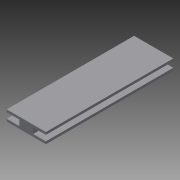
# Autodesk Inventor part: soporte fio
Saved by Autodesk Inventor 2013 (Build 170138000, 138)
## iProperties
Created: 2013-04-24
Part Number: soporte fio
Material: Generic
Document SubType Name: Modeling
Designer: otrab
Density: 1 g/cm^3
Author: otrab
Autodesk Inventor part; units mm, degrees
ref_plane "YZ Plane" through (0, 0, 0) normal (1, 0, 0) x (0, 1, 0)
ref_plane "XZ Plane" through (0, 0, 0) normal (0, 1, 0) x (-1, 0, 0)
ref_plane "XY Plane" through (0, 0, 0) normal (0, 0, 1) x (1, 0, 0)
sketch "Sketch1" plane through (0, 0, 0) normal (0, 1, 0) x (-1, 0, 0)
  line L0 (0, 0) -> (0, 1)
  line L1 (0, 1) -> (5.2, 1)
  line L2 (5.2, 1) -> (5.2, 3.3)
  line L3 (5.2, 3.3) -> (0, 3.3)
  line L4 (0, 3.3) -> (0, 4.3)
  line L5 (0, 4.3) -> (6, 4.3)
  line L6 (8, 7.1013) -> (8, -1.6755) construction
  line L7 (0, 0) -> (9, 0)
  line L8 (16, 0) -> (16, 1)
  line L9 (16, 1) -> (10.8, 1)
  line L10 (10.8, 1) -> (10.8, 3.3)
  line L11 (10.8, 3.3) -> (16, 3.3)
  line L12 (16, 3.3) -> (16, 4.3)
  line L13 (16, 4.3) -> (6, 4.3)
  line L14 (16, 0) -> (9, 0)
  dimension "d0" = 1
  dimension "d2" = 2.3
  dimension "d5" = 1
  dimension "d10" = 2.8
  dimension "d11" = 16
  dimension "d12" = 16
  constraints: 30 end point, 6 perpendicular, 6 symmetric about line, 1 parallel, 1 vertical
  measures "d0" distance of L0.start L0.end
  measures "d2" distance of L1.end L2.end
  measures "d5" distance of L3.end L4.end
  measures "d10" distance between parallel lines of L10 L6
  measures "d11" distance of L12.end L4.end
  measures "d12" distance of L14.start L0.start
extrude "Extrusion1" add sketch "Sketch1" along normal blind 52
equation "\"d12\" = d11"
body "Solid1"
